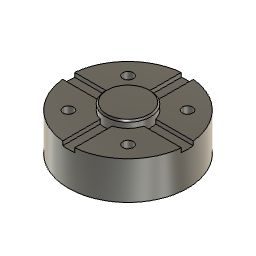
sphere_PS1_USB_C v6 (Autodesk Fusion 360 design; units mm, degrees)
Autodesk Fusion 360 part; units mm, degrees
note: some values were not read from the file. Set by a fixed rule: which sketch regions a step uses.
sketch "Skizze1" plane through (0, 0, 0) normal (0, 0, 1) x (1, 0, 0)
  circle A0 centre (0, 0) radius 20
  circle A1 centre (0, 0) radius 1.7
  line L0 (0, 23) -> (0, -24.4681) construction
  circle A2 centre (0, 0) radius 7.55
  line L1 (24, 0) -> (-23.5704, 0) construction
  line L2 (-23.8139, 10) -> (38.4686, 10) construction
  line L3 (-25.6457, -10) -> (29, -10) construction
  line L4 (-10, 25.6893) -> (-10, -22.4618) construction
  line L5 (10, 21.0661) -> (10, -25) construction
  circle A3 centre (-10, 10) radius 1.75
  circle A4 centre (10, 10) radius 1.75
  circle A5 centre (10, -10) radius 1.75
  circle A6 centre (-10, -10) radius 1.75
  line L6 (-2, 19.8997) -> (-2, -19.8997)
  line L7 (2, 19.8997) -> (2, -19.8997)
  line L8 (-19.8997, 2) -> (19.8997, 2)
  line L9 (-19.8997, -2) -> (19.8997, -2)
  point P0 (-10, 10)
  point P1 (10, 10)
  point P2 (10, -10)
  point P3 (-10, -10)
  dimension "d1" = 40
  dimension "d2" = 3.4
  dimension "d25" = 15.1
  dimension "d69" = 10
  dimension "d70" = 10
  dimension "d71" = 10
  dimension "d72" = 10
  dimension "d73" = 3.5
  dimension "d74" = 3.5
  dimension "d75" = 3.5
  dimension "d76" = 3.5
  dimension "d85" = 2
  dimension "d86" = 2
  dimension "d87" = 2
  dimension "d88" = 2
  constraint coincident A0.centre A1.centre
  constraint concentric A0 A1
  constraint vertical L0
  constraint concentric A1 A2
  constraint horizontal L1
  constraint coincident A0.centre L1
  constraint horizontal L2
  constraint horizontal L3
  constraint vertical L4
  constraint vertical L5
  constraint coincident L4 P0
  constraint coincident L2 P0
  constraint coincident L5 P1
  constraint coincident L2 P1
  constraint coincident L3 P2
  constraint coincident L5 P2
  constraint coincident L4 P3
  constraint coincident L3 P3
  constraint coincident P2 A5.centre
  constraint coincident P1 A4.centre
  constraint coincident P0 A3.centre
  constraint coincident P3 A6.centre
  constraint vertical L6
  constraint vertical L7
  constraint horizontal L8
  constraint horizontal L9
  constraint coincident A0 L7.start
  constraint coincident A0 L6.start
  constraint coincident A0 L8.start
  constraint coincident A0 L9.start
  constraint coincident A0 L8.end
  constraint coincident A0 L9.end
  constraint coincident A0 L7.end
  constraint coincident A0 L6.end
  measures "d1" diameter of A0
  measures "d2" diameter of A1
  measures "d25" diameter of A2
  measures "d69" distance of L0 L5
  measures "d70" distance of L0 L4
  measures "d71" distance of L1 L2
  measures "d72" distance of L1 L3
  measures "d73" diameter of A6
  measures "d74" diameter of A3
  measures "d75" diameter of A4
  measures "d76" diameter of A5
  measures "d85" distance of L1 L9
  measures "d86" distance of L1 L8
  measures "d87" distance of L0 L7
  measures "d88" distance of L0 L6
extrude "Extrusion1" add sketch "Skizze1" along normal blind 15 contours A2 L7 L8 | A2 L7 L8 L9 | A2 L7 L9 | A2 L6 L7 L8 | L6 L7 L8 L9 | A2 L6 L7 L9 | A2 L6 L8 | A2 L6 L8 L9 | A2 L6 L9 | A1
extrude "Extrusion2" cut sketch "Skizze1" along normal blind 14 contours A1
extrude "Extrusion5" add sketch "Skizze1" along normal blind 12.7 contours A0 A2 L7 L8 | A0 A2 L7 L9 | A0 A2 L6 L8 | A0 A2 L6 L9
extrude "Extrusion11" add sketch "Skizze1" along normal blind 11.3 contours A0 A2 L8 L9 | A0 A2 L6 L7 | A0 A2 L6 L7 | A0 A2 L8 L9
ref_plane "Arbeitsebene1" through (0, 0, 7.5) normal (0, 0, -1) x (-1, 0, 0)
sketch "Skizze2" plane through (0, 0, 7.5) normal (0, 0, -1) x (-1, 0, 0)
  line L0 (0, 19.4975) -> (0, -17.4097) construction
  line L1 (-20.2047, 0) -> (24.515, 0) construction
  line L2 (11, 10) -> (-11.3533, 10) construction
  line L3 (11, -10) -> (-11, -10) construction
  line L4 (10, 11.7482) -> (10, -12.1179) construction
  line L5 (-10, 11.5155) -> (-10, -12.3496) construction
  line L6 (11.6454, 7.15) -> (13.2909, 10)
  line L7 (13.2909, 10) -> (11.6454, 12.85)
  line L8 (11.6454, 12.85) -> (8.3546, 12.85)
  line L9 (8.3546, 12.85) -> (6.7091, 10)
  line L10 (6.7091, 10) -> (8.3546, 7.15)
  line L11 (8.3546, 7.15) -> (11.6454, 7.15)
  line L12 (-8.3546, 7.15) -> (-6.7091, 10)
  line L13 (-6.7091, 10) -> (-8.3546, 12.85)
  line L14 (-8.3546, 12.85) -> (-11.6454, 12.85)
  line L15 (-11.6454, 12.85) -> (-13.2909, 10)
  line L16 (-13.2909, 10) -> (-11.6454, 7.15)
  line L17 (-11.6454, 7.15) -> (-8.3546, 7.15)
  line L18 (-11.6454, -7.15) -> (-13.2909, -10)
  line L19 (-13.2909, -10) -> (-11.6454, -12.85)
  line L20 (-11.6454, -12.85) -> (-8.3546, -12.85)
  line L21 (-8.3546, -12.85) -> (-6.7091, -10)
  line L22 (-6.7091, -10) -> (-8.3546, -7.15)
  line L23 (-8.3546, -7.15) -> (-11.6454, -7.15)
  line L24 (8.3546, -7.15) -> (6.7091, -10)
  line L25 (6.7091, -10) -> (8.3546, -12.85)
  line L26 (8.3546, -12.85) -> (11.6454, -12.85)
  line L27 (11.6454, -12.85) -> (13.2909, -10)
  line L28 (13.2909, -10) -> (11.6454, -7.15)
  line L29 (11.6454, -7.15) -> (8.3546, -7.15)
  point P0 (10, 10)
  point P1 (-10, 10)
  point P2 (-10, -10)
  point P3 (10, -10)
  dimension "d77" = 10
  dimension "d78" = 10
  dimension "d79" = 10
  dimension "d80" = 10
  dimension "d81" = 5.7
  dimension "d82" = 5.7
  dimension "d83" = 5.7
  dimension "d84" = 5.7
  constraint vertical L0
  constraint coincident L0 origin
  constraint horizontal L1
  constraint coincident L1 origin
  constraint horizontal L2
  constraint horizontal L3
  constraint parallel L0 L4
  constraint perpendicular L3 L5
  constraint coincident L2 P0
  constraint coincident L4 P0
  constraint coincident L5 P1
  constraint coincident L2 P1
  constraint coincident L3 P2
  constraint coincident L5 P2
  constraint coincident L4 P3
  constraint coincident L3 P3
  measures "d77" distance of L0 L5
  measures "d78" distance of L0 L4
  measures "d79" distance of L1 L2
  measures "d80" distance of L1 L3
  measures "d81" distance of L8 L11
  measures "d82" distance of L14 L17
  measures "d83" distance of L20 L23
  measures "d84" distance of L26 L29
extrude "Extrusion4" cut sketch "Skizze2" along normal blind 2.6
chamfer "Fase2" distance 0.5 angle 45 1 edges at (-7.0391, -2.7302, 15)
